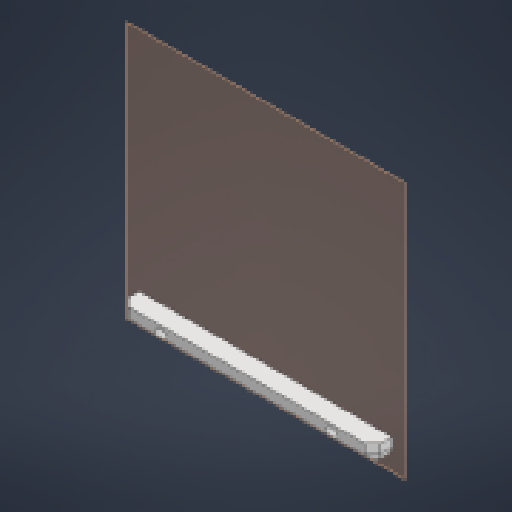
# Autodesk Inventor part: front_case_buttons
Saved by Autodesk Inventor 2024 (Build 280153000, 153)
## iProperties
Created: 2026-07-02
Part Number: front_case_buttons
Material: Generic
Document SubType Name: Modeling
Designer: schar
Density: 1 g/cm^3
Appearance: Default
Author: schar
Autodesk Inventor part; units mm, degrees
ref_plane "YZ Plane" through (0, 0, 0) normal (1, 0, 0) x (0, 1, 0)
ref_plane "XZ Plane" through (0, 0, 0) normal (0, 1, 0) x (-1, 0, 0)
ref_plane "XY Plane" through (0, 0, 0) normal (0, 0, 1) x (1, 0, 0)
ref_plane "Work Plane1" through (0, 0, 0) normal (0, 0, 1) x (1, 0, 0)
sketch "Sketch1" plane through (0, 0, 0) normal (0, 0, 1) x (1, 0, 0)
  arc A0 (154.69, -45.76) -> (149.66, -40.73) centre (149.66, -45.76) ccw projected
  line L0 (80.43, -40.73) -> (149.66, -40.73) projected
  arc A1 (80.43, -40.73) -> (75.4, -45.76) centre (80.43, -45.76) ccw projected
  line L1 (75.4, -56.1) -> (75.4, -45.76) projected
  line L2 (75.4, -111.15) -> (75.4, -56.1) projected
  arc A2 (75.4, -111.15) -> (78.35, -114.1) centre (78.35, -111.15) ccw projected
  line L3 (151.75, -114.1) -> (78.35, -114.1) projected
  arc A3 (151.75, -114.1) -> (154.7, -111.15) centre (151.75, -111.15) ccw projected
  line L4 (154.7, -56.1) -> (154.7, -111.15) projected
  line L5 (154.69, -45.76) -> (154.7, -56.1) projected
  circle A4 centre (88.35, -111.15) radius 2 projected
  circle A5 centre (85.05, -103.33) radius 0.85 projected
  circle A6 centre (85.05, -98.25) radius 2 projected
  circle A7 centre (90.13, -100.79) radius 0.75 projected
  circle A8 centre (105.05, -103.33) radius 0.85 projected
  circle A9 centre (105.05, -98.25) radius 2 projected
  circle A10 centre (110.13, -100.79) radius 0.75 projected
  circle A11 centre (85.05, -93.17) radius 0.85 projected
  circle A12 centre (87.59, -94.44) radius 0.75 projected
  circle A13 centre (78.45, -86.75) radius 0.75 projected
  circle A14 centre (78.45, -84.65) radius 0.45 projected
  circle A15 centre (78.45, -82.65) radius 0.45 projected
  circle A16 centre (86.05, -83) radius 1.05 projected
  circle A17 centre (78.45, -80.65) radius 0.45 projected
  circle A18 centre (78.45, -78.55) radius 0.75 projected
  circle A19 centre (85.5, -78.88) radius 0.5 projected
  circle A20 centre (95.11, -86.5) radius 1.5 projected
  circle A21 centre (90.11, -81.1) radius 0.5 projected
  circle A22 centre (93.81, -81.1) radius 0.5 projected
  circle A23 centre (105.05, -93.17) radius 0.85 projected
  circle A24 centre (107.59, -94.44) radius 0.75 projected
  circle A25 centre (125.05, -103.33) radius 0.85 projected
  circle A26 centre (130.13, -100.79) radius 0.75 projected
  circle A27 centre (125.05, -98.25) radius 2 projected
  circle A28 centre (141.75, -111.15) radius 2 projected
  circle A29 centre (145.05, -103.33) radius 0.85 projected
  circle A30 centre (150.13, -100.79) radius 0.75 projected
  circle A31 centre (145.05, -98.25) radius 2 projected
  circle A32 centre (127.59, -94.44) radius 0.75 projected
  circle A33 centre (125.05, -93.17) radius 0.85 projected
  circle A34 centre (145.05, -93.17) radius 0.85 projected
  circle A35 centre (147.59, -94.44) radius 0.75 projected
  circle A36 centre (135, -86.5) radius 1.5 projected
  circle A37 centre (143.95, -83) radius 1.05 projected
  circle A38 centre (85.5, -76.34) radius 0.5 projected
  circle A39 centre (85.5, -73.8) radius 0.5 projected
  circle A40 centre (85.5, -71.26) radius 0.5 projected
  circle A41 centre (85.5, -68.72) radius 0.5 projected
  circle A42 centre (85.5, -66.18) radius 0.5 projected
  circle A43 centre (85.5, -63.64) radius 0.5 projected
  circle A44 centre (85.5, -61.1) radius 0.5 projected
  circle A45 centre (86.05, -57.2) radius 1.05 projected
  circle A46 centre (80.4, -50.93) radius 2 projected
  arc A47 (90, -44) -> (90, -48) centre (90, -46) ccw projected
  line L6 (100, -44) -> (90, -44) projected
  arc A48 (100, -48) -> (100, -44) centre (100, -46) ccw projected
  line L7 (90, -48) -> (100, -48) projected
  circle A49 centre (115.05, -46) radius 3 projected
  circle A50 centre (143.95, -57.2) radius 1.05 projected
  arc A51 (130.1, -44) -> (130.1, -48) centre (130.1, -46) ccw projected
  line L8 (140.1, -44) -> (130.1, -44) projected
  arc A52 (140.1, -48) -> (140.1, -44) centre (140.1, -46) ccw projected
  line L9 (130.1, -48) -> (140.1, -48) projected
  circle A53 centre (149.695, -50.93) radius 2 projected
  line L10 (93.0123, -107.25) -> (77.0877, -107.25) projected
  line L11 (75.4, -108.2757) -> (154.7, -108.2757)
  point P0 (0, 0)
  constraints: 2 end point, 2 point on line, 1 perpendicular
extrude "Extrusion1" add sketch "Sketch1" along normal blind 6 contours L4 A3 L3 A2 L2 L11
chamfer "Chamfer1" distance 2.5 angle 45 5 edges at (115.05, -114.1, 6) (153.836, -113.236, 6) (154.7, -109.7129, 6) (76.264, -113.236, 6) (75.4, -109.7129, 6)
sketch "Sketch2" plane through (0, 0, 6) normal (0, 0, 1) x (1, 0, 0)
  arc A0 (90.2987, -111.6) -> (86.4013, -111.6) centre (88.35, -111.15) ccw projected
  circle A1 centre (88.35, -111.15) radius 4.25
  circle A2 centre (141.75, -111.15) radius 2 projected
  circle A3 centre (141.75, -111.15) radius 4.25
  arc A4 (86.4013, -111.6) -> (90.2987, -111.6) centre (88.35, -111.15) ccw projected
  point P0 (0, 0)
  dimension "d5" = 8.5
  dimension "d6" = 8.5
  constraints: 2 centre point, 2 coincident
  measures "d5" diameter of A1
  measures "d6" diameter of A3
extrude "Extrusion2" cut sketch "Sketch2" against normal blind 3
body "Solid1"
